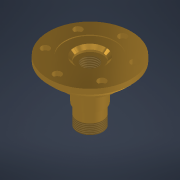
# Autodesk Inventor part: Tuerca2
Saved by Autodesk Inventor 2022 (Build 260153000, 153)
## iProperties
Created: 2021-09-12
Part Number: Tuerca2
Material: Brass, Soft Yellow
Document SubType Name: Modeling
Designer: Andres
Density: 8.47 g/cm^3
Appearance: Brass - Satin
Author: Andres
Autodesk Inventor part; units mm, degrees
ref_plane "YZ Plane" through (0, 0, 0) normal (1, 0, 0) x (0, 1, 0)
ref_plane "XZ Plane" through (0, 0, 0) normal (0, 1, 0) x (-1, 0, 0)
ref_plane "XY Plane" through (0, 0, 0) normal (0, 0, 1) x (1, 0, 0)
sketch "Sketch1" plane through (0, 0, 0) normal (1, 0, 0) x (0, 1, 0)
  line L0 (50, -8) -> (50, -41)
  line L1 (50, -41) -> (40, -41)
  line L2 (30.4606, -25) -> (30.4606, -14)
  line L3 (30.4606, -14) -> (0, -14)
  line L4 (0, -14) -> (0, -8)
  line L5 (0, -8) -> (50, -8)
  line L6 (260.8418, 0) -> (-144.0727, 0)
  line L7 (49, -25) -> (49, -12.5)
  line L8 (49, -12.5) -> (44, -12.5)
  line L9 (44, -12.5) -> (44, -8)
  line L10 (40, -25) -> (40, -41)
  line L11 (40, -25) -> (30.4606, -25)
  line L12 (49, -25) -> (50, -25)
  line L13 (30.4606, 22.9) -> (30.4606, -22.9) projected
  line L14 (10, -8) -> (10, -14)
  point P0 (0, 0)
  point P1 (0, -11)
  dimension "d3" = 28
  dimension "d4" = 50
  dimension "d10" = 16
  dimension "d11" = 82
  dimension "d13" = 25
  dimension "d14" = 50
  dimension "d15" = 1
  dimension "d16" = 6
  dimension "d21" = 10
  dimension "d23" = 50
  dimension "d54" = 10
  constraints: 29 end point, 6 perpendicular, 5 point on line, 4 vertical, 2 horizontal, 1 collinear, 1 midpoint, 1 parallel, 1 vertical alignment
  measures "d3" diameter of L3 L6
  measures "d4" distance between parallel lines of L0 L4
  measures "d10" diameter of L5 L6
  measures "d11" diameter of L1 L6
  measures "d13" diameter of L8 L6
  measures "d14" diameter of L7.start L6
  measures "d15" distance between parallel lines of L0 L7
  measures "d16" distance between parallel lines of L0 L9
  measures "d21" distance between parallel lines of L0 L10
  measures "d23" diameter of L11 L6
  measures "d54" distance between parallel lines of L4 L14
revolve "Revolution1" add sketch "Sketch1" angle 360 about axis through (0, 260.8418, 0) along (0, -1, 0) contours L0 L1 L10 L11 L2 L13 L5 L9 L8 L7 L12 | L13 L3 L14 L5
thread "Thread1" size "M16x2" class "6H" standard "ANSI Metric M Profile" length 44
chamfer "Chamfer1" distance 5 angle 45 1 edges at (0, 40, 41)
chamfer "Chamfer2" distance 5 angle 45 1 edges at (0, 40, 25)
sketch "Sketch2" plane through (0, 50, 0) normal (0, 1, 0) x (1, 0, 0)
  circle A0 centre (0, 0) radius 8 construction
  circle A1 centre (0, 0) radius 32.5 construction
  point P0 (0, 0)
  point P1 (0, -32.5)
  point P2 (28.1458, -16.25)
  point P3 (28.1458, 16.25)
  point P4 (0, 32.5)
  point P5 (-28.1458, 16.25)
  point P6 (-28.1458, -16.25)
  dimension "d30" = 65
  dimension "d33" = 360
  constraints: 2 vertical alignment, 1 coincident, 9 other
hole "Hole1" at (0, 50, 32.5) at (28.1458, 50, 16.25) at (28.1458, 50, -16.25) at (0, 50, -32.5) at (-28.1458, 50, -16.25) at (-28.1458, 50, 16.25) direction (0, -1, 0) diameter 4.5 depth 10 tip angle 118 counterbore diameter 8 counterbore depth 4.6 clearance for "Socket Head Cap Screw ISO 4762" size "M4" standard "ISO"
chamfer "Chamfer4" distance 3 angle 45 1 edges at (0, 49, 12.5)
sketch "Sketch3" plane through (0, 10, 0) normal (0, -1, 0) x (1, 0, 0)
  circle A0 centre (0, 0) radius 14 projected
  circle A1 centre (0, 0) radius 8 projected
  circle A2 centre (0, 0) radius 12.5
  circle A3 centre (0, 0) radius 10
  point P0 (0, 0)
  dimension "d45" = 25
  dimension "d48" = 20
  constraints: 2 centre point, 2 coincident
  measures "d45" diameter of A2
  measures "d48" diameter of A3
extrude "Extrusion1" add sketch "Sketch3" along normal blind 20 contours A2
chamfer "Chamfer5" distance 2 angle 45 1 edges at (-10, 10, 0)
thread "Thread2" size "M25x1.5" class "6g" standard "ANSI Metric M Profile" length 10
body "Solid1"
